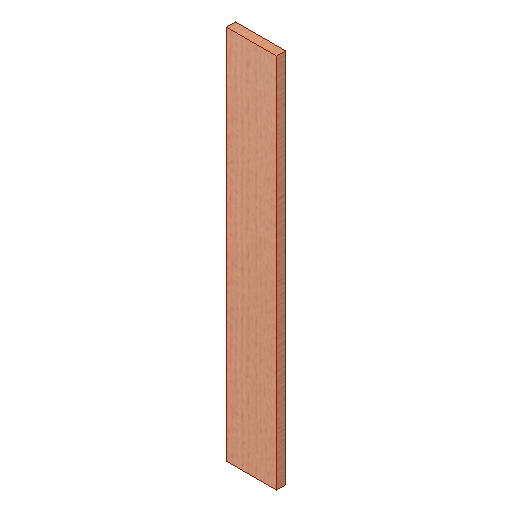
# Autodesk Inventor part: CNCM_WOOD_18mm_Base_plate_reinforcement
Saved by Autodesk Inventor 2025 (Build 290162010, 162A)
## iProperties
Created: 2018-07-30
Part Number: CNCM_WOOD_18mm_Base_plate_reinforcement
Material: Generic
Document SubType Name: Modeling
Designer: Andrzej
Density: 1 g/cm^3
Appearance: White Oak - Natural Medium Gloss
Author: Andrzej
Autodesk Inventor part; units mm, degrees
ref_plane "YZ Plane" through (0, 0, 0) normal (1, 0, 0) x (0, 1, 0)
ref_plane "XZ Plane" through (0, 0, 0) normal (0, 1, 0) x (-1, 0, 0)
ref_plane "XY Plane" through (0, 0, 0) normal (0, 0, 1) x (1, 0, 0)
sketch "Sketch1" plane through (0, 0, 0) normal (0, 0, 1) x (1, 0, 0)
  line L0 (-53.8093, 745.2918) -> (46.1907, 745.2918)
  line L1 (46.1907, 745.2918) -> (46.1907, -4.7082)
  line L2 (46.1907, -4.7082) -> (-53.8093, -4.7082)
  line L3 (-53.8093, -4.7082) -> (-53.8093, 745.2918)
  point P0 (0, 0)
  dimension "d0" = 100
  dimension "d1" = 750
  constraints: 8 end point, 2 parallel, 1 horizontal, 1 perpendicular
  measures "d0" distance of L1.end L2.end
  measures "d1" distance of L0.end L1.end
extrude "Extrusion1" add sketch "Sketch1" along normal blind 18
body "Solid1"
